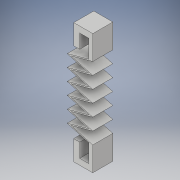
# Autodesk Inventor part: Spring Mk 1.1
Saved by Autodesk Inventor 2019 (Build 230136000, 136)
## iProperties
Created: 2019-02-23
Part Number: Spring Mk 1.1
Material: Generic
Document SubType Name: Modeling
Designer: Kepler
Density: 1 g/cm^3
Appearance: Default
Author: Kepler
Autodesk Inventor part; units mm, degrees
ref_plane "YZ Plane" through (0, 0, 0) normal (1, 0, 0) x (0, 1, 0)
ref_plane "XZ Plane" through (0, 0, 0) normal (0, 1, 0) x (-1, 0, 0)
ref_plane "XY Plane" through (0, 0, 0) normal (0, 0, 1) x (1, 0, 0)
sketch "Sketch2" plane through (0, 0, 0) normal (0, 0, 1) x (1, 0, 0)
  line L0 (0, 0) -> (0, 5)
  line L1 (0, 5) -> (1.5, 5)
  line L2 (0, 0) -> (4.75, 0)
  line L3 (4.75, 0) -> (4.75, 6)
  line L4 (1.5, 5) -> (1.5, 1.5)
  line L5 (1.5, 1.5) -> (3.75, 1.5)
  line L6 (3.75, 1.5) -> (3.75, 6)
  line L7 (3.75, 6) -> (-1.6323, 7.5)
  line L8 (-1.6323, 7.5) -> (3.75, 9)
  line L9 (4.75, 6) -> (-0.6323, 7.5)
  line L10 (-0.6323, 7.5) -> (4.75, 9)
  line L11 (4.75, 9) -> (-0.6323, 10.5)
  line L12 (3.75, 9) -> (-1.6323, 10.5)
  line L13 (-1.6323, 10.5) -> (3.75, 12)
  line L14 (-0.6323, 10.5) -> (4.75, 12)
  line L15 (4.75, 12) -> (-0.6323, 13.5)
  line L16 (3.75, 12) -> (-1.6323, 13.5)
  line L17 (-1.6323, 13.5) -> (3.75, 15)
  line L18 (-0.6323, 13.5) -> (4.75, 15)
  line L19 (4.75, 15) -> (-0.6323, 16.5)
  line L20 (3.75, 15) -> (-1.6323, 16.5)
  line L21 (-1.6323, 16.5) -> (3.75, 18)
  line L22 (-0.6323, 16.5) -> (4.75, 18)
  line L23 (4.75, 18) -> (-0.6323, 19.5)
  line L24 (3.75, 18) -> (-1.6323, 19.5)
  line L25 (-1.6323, 19.5) -> (3.75, 21)
  line L26 (-0.6323, 19.5) -> (4.75, 21)
  line L27 (4.75, 21) -> (-0.6323, 22.5)
  line L28 (3.75, 21) -> (-1.6323, 22.5)
  line L29 (-1.6323, 22.5) -> (3.75, 24)
  line L30 (-0.6323, 22.5) -> (4.75, 24)
  line L31 (5.9357, 15) -> (7.813, 15) construction
  line L32 (0, 30) -> (0, 25)
  line L33 (0, 25) -> (1.5, 25)
  line L34 (0, 30) -> (4.75, 30)
  line L35 (4.75, 30) -> (4.75, 24)
  line L36 (1.5, 25) -> (1.5, 28.5)
  line L37 (1.5, 28.5) -> (3.75, 28.5)
  line L38 (3.75, 28.5) -> (3.75, 24)
  dimension "d14" = 5
  dimension "d15" = 1.5
  dimension "d16" = 4.75
  dimension "d17" = 6
  dimension "d18" = 3.5
  dimension "d19" = 2.25
  dimension "d24" = 4.5
  dimension "d25" = 3
  dimension "d28" = 1.5
  dimension "d29" = 0
  dimension "d37" = 15.573
  dimension "d38" = 15
  dimension "d39" = 3.063
  dimension "d40" = 1.1857
  constraints: 78 end point, 6 symmetric about line, 4 parallel, 4 perpendicular, 2 horizontal, 2 vertical
  measures "d14" distance of L0.start L0.end
  measures "d15" distance of L0.end L1.end
  measures "d16" distance of L0.start L2.end
  measures "d17" distance of L2.end L3.end
  measures "d18" distance of L1.end L4.end
  measures "d19" distance of L4.end L5.end
  measures "d24" distance of L5.end L6.end
  measures "d25" distance of L10.end L3.end
  measures "d28" vertical distance of L3.end L9.end
  measures "d29" distance from line of L10.end L3
  measures "d37" angle of L30 L31
  measures "d38" distance between parallel lines of L34 L31
  measures "d39" distance from line of L31.end L35
  measures "d40" distance from line of L31.start L35
extrude "Extrusion2" add sketch "Sketch2" along normal blind 5
equation "\"d28\" = 0.5 * d25"
body "Solid2"
